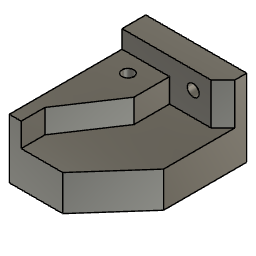
obj1 (Autodesk Fusion 360 design; units mm, degrees)
Autodesk Fusion 360 part; units mm, degrees
sketch "Sketch1" plane through (0, 0, 0) normal (0, 0, 1) x (1, 0, 0) in component "Base"
  line L0 (-85, -115) -> (-85, 115)
  line L1 (-85, 115) -> (85, 115)
  line L2 (85, -115) -> (-85, 115) construction
  line L3 (-85, -115) -> (85, 115) construction
  line L4 (-85, -115) -> (-85, 115)
  line L5 (85, 115) -> (85, -25)
  line L6 (-85, -115) -> (5, -115)
  line L7 (85, -25) -> (5, -115)
  dimension "d1" = 170
  dimension "d2" = 230
  dimension "d3" = 140
  dimension "d4" = 90
  constraint coincident L2 origin
  constraint coincident L3 origin
  constraint perpendicular L1 L5
  constraint perpendicular L4 L6
  measures "d1" distance of L0.end L1.end
  measures "d2" distance of L0.start L0.end
  measures "d3" distance of L1.end L5.end
  measures "d4" distance of L0.start L6.end
extrude "Extrude1" add sketch "Sketch1" along normal blind 60 in component "Base"
sketch "Sketch2" plane through (0, 0, 60) normal (0, 0, 1) x (-1, 0, 0) in component "Base"
  line L0 (85, 115) -> (-5, 115)
  line L1 (-5, 115) -> (-85, 25)
  line L2 (-85, 25) -> (-85, -115)
  line L3 (-85, -115) -> (85, -115)
  line L4 (85, -115) -> (85, 115)
  line L5 (-85, -115) -> (-85, -95)
  line L6 (85, -115) -> (85, -75)
  line L7 (85, -75) -> (-65, -75)
  line L8 (-65, -75) -> (-85, -95)
  dimension "d7" = 20
  dimension "d8" = 40
  dimension "d9" = 150
  constraint coincident L2.end L3.start
  constraint perpendicular L3 L5
  constraint coincident L3.end L4.start
  constraint perpendicular L3 L6
  constraint perpendicular L6 L7
  measures "d7" distance of L2.end L5.end
  measures "d8" distance of L3.end L6.end
  measures "d9" distance of L6.end L7.end
extrude "Extrude2" add sketch "Sketch2" along normal blind 70 contours L2 L3 L4 L5 L6 L7 L8 in component "Base"
sketch "Sketch3" plane through (0, 0, 60) normal (0, 0, 1) x (-1, 0, 0) in component "Base"
  line L0 (-65, -75) -> (85, -75)
  line L1 (85, -75) -> (85, 115)
  line L2 (85, 115) -> (-5, 115)
  line L3 (-5, 115) -> (-85, 25)
  line L4 (-85, 25) -> (-85, -95)
  line L5 (-85, -95) -> (-65, -75)
  line L6 (85, -75) -> (85, 115)
  line L7 (85, 115) -> (65, 115)
  line L8 (65, 115) -> (65, 75)
  line L9 (85, -75) -> (5, -75)
  line L10 (5, -75) -> (5, -15)
  line L11 (5, -15) -> (65, 75)
  dimension "d12" = 20
  dimension "d13" = 40
  dimension "d14" = 80
  dimension "d15" = 60
  constraint coincident L0.end L1.start
  constraint coincident L1.end L2.start
  constraint perpendicular L6 L7
  constraint perpendicular L7 L8
  constraint perpendicular L6 L9
  constraint perpendicular L9 L10
  measures "d12" distance of L1.end L7.end
  measures "d13" distance of L7.end L8.end
  measures "d14" distance of L0.end L9.end
  measures "d15" distance of L9.end L10.end
extrude "Extrude3" add sketch "Sketch3" along normal blind 40 contours L0 L1 L2 L6 L7 L8 L9 L10 L11 in component "Base"
sketch "Sketch4" plane through (0, 75, 0) normal (0, -1, 0) x (1, 0, 0) in component "Base"
  line L0 (-5, 100) -> (-5, 60)
  line L1 (-5, 60) -> (65, 60)
  line L2 (65, 60) -> (65, 130)
  line L3 (65, 130) -> (-85, 130)
  line L4 (-85, 130) -> (-85, 100)
  line L5 (-85, 100) -> (-5, 100)
  line L6 (65, 130) -> (25, 130)
  line L7 (65, 130) -> (35, 130)
  line L8 (65, 130) -> (65, 100)
  circle A0 centre (35, 100) radius 10
  dimension "d19" = 30
  constraint coincident L2.end L3.start
  constraint perpendicular L2 L6
  constraint perpendicular L2 L7
  constraint coincident L2 L8.end
  constraint perpendicular L6 L8
  measures "d19" distance of L2.end L7.end
extrude "Extrude4" cut sketch "Sketch4" against normal up to surface (40 mm away) contours A0 in component "Base"
sketch "Sketch5" plane through (0, 0, 100) normal (0, 0, 1) x (-1, 0, 0) in component "Base"
  line L0 (85, -75) -> (85, 115)
  line L1 (85, 115) -> (65, 115)
  line L2 (65, 115) -> (65, 75)
  line L3 (65, 75) -> (5, -15)
  line L4 (5, -15) -> (5, -75)
  line L5 (5, -75) -> (85, -75)
  line L6 (85, -75) -> (45, -75)
  line L7 (85, -75) -> (85, -45)
  circle A0 centre (45, -45) radius 10
  dimension "d22" = 30
  dimension "d23" = 20
  constraint coincident L0.start L5.end
  constraint midpoint L5 L6.end
  constraint perpendicular L6 L7
  measures "d22" distance of L0.start L7.end
  measures "d23" diameter of A0
extrude "Extrude5" cut sketch "Sketch5" against normal up to surface (100 mm away) contours A0 in component "Base"
component "Base" placed x (1, 0, 0) y (0, 1, 0) z (0, 0, 1) at (0, 0, 0)
